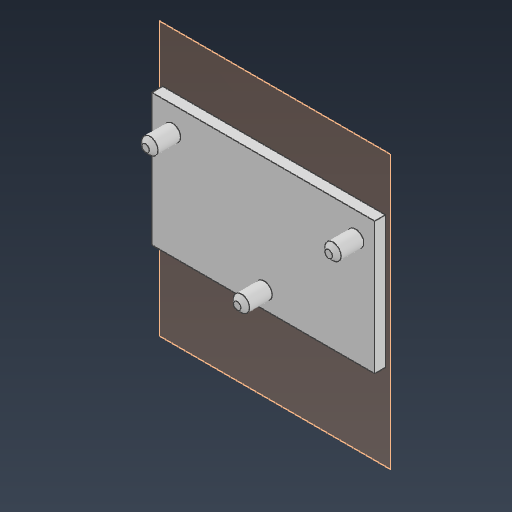
# Autodesk Inventor part: vesc_holes_check
Saved by Autodesk Inventor 2023 (Build 270158000, 158)
## iProperties
Created: 2025-12-26
Part Number: vesc_holes_check
Material: Generic
Document SubType Name: Modeling
Designer: szymo
Density: 1 g/cm^3
Appearance: Default
Author: szymo
Autodesk Inventor part; units mm, degrees
ref_plane "YZ Plane" through (0, 0, 0) normal (1, 0, 0) x (0, 1, 0)
ref_plane "XZ Plane" through (0, 0, 0) normal (0, 1, 0) x (-1, 0, 0)
ref_plane "XY Plane" through (0, 0, 0) normal (0, 0, 1) x (1, 0, 0)
ref_plane "Work Plane3" through (6.1355, -21.1735, -7.3328) normal (0, 0, 1) x (1, 0, 0)
sketch "Sketch3" plane through (6.1355, -21.1735, -7.3328) normal (0, 0, 1) x (1, 0, 0)
  line L0 (20.5093, -9.3897) -> (-20.8066, -9.3897)
  line L1 (-20.8066, -9.3897) -> (-20.8066, 15.1082)
  line L2 (-20.8066, 15.1082) -> (20.5093, 15.1082)
  line L3 (20.5093, 15.1082) -> (20.5093, -9.3897)
  line L4 (-12.3, 2) -> (7, 2) projected
  circle A0 centre (16.975, 10.575) radius 1.621 projected
  circle A1 centre (0, -6.25) radius 1.621 projected
  circle A2 centre (-16.975, 10.575) radius 1.621 projected
  line L5 (-19.5, 23) -> (-19.5, -23) projected
  line L6 (-19.5, -23) -> (-13.8, -23) projected
  line L7 (-13.8, -23) -> (-13.8, -17.4) projected
  arc A3 (-10.8, -14.4) -> (-13.8, -17.4) centre (-10.8, -17.4) ccw projected
  line L8 (-10.8, -14.4) -> (10.8, -14.4) projected
  arc A4 (13.8, -17.4) -> (10.8, -14.4) centre (10.8, -17.4) ccw projected
  line L9 (13.8, -17.4) -> (13.8, -23) projected
  line L10 (13.8, -23) -> (19.5, -23) projected
  line L11 (19.5, -23) -> (19.5, 23) projected
  line L12 (19.5, 23) -> (-19.5, 23) projected
  circle A5 centre (-17, -20) radius 1.25 projected
  circle A6 centre (17, -20) radius 1.25 projected
  circle A7 centre (17, 20) radius 1.25 projected
  circle A8 centre (-17, 20) radius 1.25 projected
  circle A9 centre (0, -6.25) radius 1.5
  circle A10 centre (16.975, 10.575) radius 1.5
  circle A11 centre (-16.975, 10.575) radius 1.5
  point P0 (-6.1355, 21.1735)
  dimension "d18" = 3
  dimension "d19" = 3
  dimension "d20" = 3
  constraints: 8 end point, 3 centre point, 3 coincident, 2 parallel, 1 horizontal, 1 perpendicular
  measures "d18" diameter of A9
  measures "d19" diameter of A10
  measures "d20" diameter of A11
extrude "Extrusion3" add sketch "Sketch3" along normal blind 2 contours L0 L11 L2 L3 | L0 L5 L2 L11 | L0 L1 L2 L5 | A0 | A1 | A2 | A9 | A10 | A11
sketch "Sketch4" plane through (6.1355, -21.1735, -5.3328) normal (0, 0, 1) x (1, 0, 0)
  circle A0 centre (16.975, 10.575) radius 1.621 projected
  circle A1 centre (0, -6.25) radius 1.621 projected
  circle A2 centre (-16.975, 10.575) radius 1.621 projected
  line L0 (-19.5, 23) -> (-19.5, -23) projected
  line L1 (-19.5, -23) -> (-13.8, -23) projected
  line L2 (-13.8, -23) -> (-13.8, -17.4) projected
  arc A3 (-10.8, -14.4) -> (-13.8, -17.4) centre (-10.8, -17.4) ccw projected
  line L3 (-10.8, -14.4) -> (10.8, -14.4) projected
  arc A4 (13.8, -17.4) -> (10.8, -14.4) centre (10.8, -17.4) ccw projected
  line L4 (13.8, -17.4) -> (13.8, -23) projected
  line L5 (13.8, -23) -> (19.5, -23) projected
  line L6 (19.5, -23) -> (19.5, 23) projected
  line L7 (19.5, 23) -> (-19.5, 23) projected
  circle A5 centre (-17, -20) radius 1.25 projected
  circle A6 centre (17, -20) radius 1.25 projected
  circle A7 centre (17, 20) radius 1.25 projected
  circle A8 centre (-17, 20) radius 1.25 projected
  circle A9 centre (0, -6.25) radius 1.5
  circle A10 centre (-16.975, 10.575) radius 1.5
  circle A11 centre (16.975, 10.575) radius 1.5
  point P0 (-6.1355, 21.1735)
  dimension "d23" = 3
  dimension "d24" = 3
  dimension "d25" = 3
  constraints: 3 centre point, 3 coincident
  measures "d23" diameter of A9
  measures "d24" diameter of A10
  measures "d25" diameter of A11
extrude "Extrusion4" add sketch "Sketch4" along normal blind 5 contours A9 | A10 | A11
chamfer "Chamfer2" distance 0.8 angle 45 3 edges at (21.6105, -10.5985, -0.3328) (4.6355, -27.4235, -0.3328) (-12.3395, -10.5985, -0.3328)
body "Solid2"
